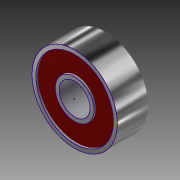
# Autodesk Inventor part: bearing
Saved by Autodesk Inventor 2014 SP2 (Build 180246200, 246)
## iProperties
Created: 2019-05-12
Part Number: bearing
Material: Generic
Document SubType Name: Modeling
Designer: GauchoHP
Density: 1 g/cm^3
Appearance: Default
Author: GauchoHP
Autodesk Inventor part; units mm, degrees
ref_plane "YZ Plane" through (0, 0, 0) normal (1, 0, 0) x (0, 1, 0)
ref_plane "XZ Plane" through (0, 0, 0) normal (0, 1, 0) x (-1, 0, 0)
ref_plane "XY Plane" through (0, 0, 0) normal (0, 0, 1) x (1, 0, 0)
sketch "Sketch1" plane through (0, 0, 0) normal (0, 1, 0) x (-1, 0, 0)
  circle A0 centre (0, 0) radius 4
  circle A1 centre (0, 0) radius 5
  circle A2 centre (0, 0) radius 11
  circle A3 centre (0, 0) radius 10
  dimension "d0" = 8
  dimension "d1" = 10
  dimension "d2" = 22
  dimension "d3" = 20
  constraints: 4 centre point, 4 coincident
  measures "d0" diameter of A0
  measures "d1" diameter of A1
  measures "d2" diameter of A2
  measures "d3" diameter of A3
extrude "Extrusion1" add sketch "Sketch1" along normal blind 7.5 contours A3
extrude "Extrusion2" add sketch "Sketch1" along normal blind 8 contours A2
extrude "Extrusion3" cut sketch "Sketch1" along normal blind 0.5 contours A3
extrude "Extrusion4" add sketch "Sketch1" along normal blind 8 contours A1
body "Solid1"
